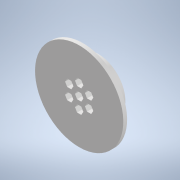
# Autodesk Inventor part: tire vtulka2
Saved by Autodesk Inventor 2022 (Build 260153000, 153)
## iProperties
Created: 2023-02-08
Part Number: tire vtulka2
Material: Типовые
Document SubType Name: Modeling
Designer: akapu
Density: 1 g/cm^3
Appearance: По умолчанию
Author: akapu
Autodesk Inventor part; units mm, degrees
ref_plane "YZ Plane" through (0, 0, 0) normal (1, 0, 0) x (0, 1, 0)
ref_plane "XZ Plane" through (0, 0, 0) normal (0, 1, 0) x (-1, 0, 0)
ref_plane "XY Plane" through (0, 0, 0) normal (0, 0, 1) x (1, 0, 0)
sketch "Эскиз1" plane through (0, 0, 0) normal (1, 0, 0) x (0, 1, 0)
  line L0 (-3.98, -3) -> (-3.38, 0)
  line L1 (-3.98, -3) -> (-56.02, -3) projected
  line L2 (-4.48, -22.93) -> (-4.48, -3)
  line L3 (-55.52, -22.93) -> (-55.52, -3)
  line L4 (-3.98, -3) -> (-56.02, -3) projected
  line L5 (-56.02, -3) -> (-56.62, 0)
  line L6 (-60, 0) -> (0, 0) projected
  line L7 (-60, 0) -> (-60, -22.93)
  line L8 (0, 0) -> (0, -22.93)
  line L9 (-60, -22.93) -> (0, -22.93) projected
  line L10 (-3.98, -3) -> (-3.98, -3)
  line L11 (-3.98, -3) -> (-3.38, 0)
  line L12 (-56.02, -3) -> (-56.02, -3)
  line L13 (-56.02, -3) -> (-56.62, 0)
  line L14 (-3.38, 0) -> (4.62, 0)
  line L15 (-56.62, 0) -> (-64.62, 0)
  line L16 (-64.62, 0) -> (-64.62, 3)
  line L17 (-64.62, 3) -> (4.62, 3)
  line L18 (4.62, 3) -> (4.62, 0)
  line L19 (-30, -3) -> (-51.25, -3)
  line L20 (-51.25, -3) -> (-8.75, -3)
  line L21 (-8.75, -3) -> (-8.75, -22.93)
  line L22 (-51.25, -3) -> (-51.25, -22.93)
  line L23 (-52.5, -22.93) -> (-51.25, -22.93)
  line L24 (-51.5625, -21.93) -> (-51.5625, -22.93)
  line L25 (-51.875, -21.93) -> (-51.25, -21.93)
  line L26 (-52.5, -22.93) -> (-51.25, -20.93)
  spline S0 degree 2 poles (-52.5, -22.93) (-51.1297, -22.7543) (-51.25, -20.93) knots 0 0 0 1 1 1
  line L27 (-8.75, -19) -> (-8.75, -12)
  line L28 (-8.75, -12) -> (-51.25, -12)
  line L29 (-30, 3) -> (-30, -22.93)
  line L30 (-8.75, -12) -> (-11.75, -12)
  line L31 (-30, -12) -> (-30, -14)
  line L32 (-11.75, -12) -> (-13.75, -14)
  line L33 (-11.75, -12) -> (-8.9216, -12) construction
  line L34 (-13.75, -14) -> (-30, -14)
  line L35 (2, 0) -> (0, 0)
  line L36 (-7.75, -4.6) -> (-8.75, -4.6)
  line L37 (-8.25, -4.6) -> (-8.25, -3)
  line L38 (-6.75, -3) -> (-8.75, -3)
  line L39 (-6.75, -3) -> (-8.75, -6.2)
  spline S1 degree 2 poles (-6.75, -3) (-8.9425, -3.2811) (-8.75, -6.2) knots 0 0 0 1 1 1
  spline S2 degree 2 poles (-53.25, -3) (-51.0575, -3.2811) (-51.25, -6.2) knots 0 0 0 1 1 1
  line L40 (-30, -14) -> (-25, -14)
  line L41 (-25, -14) -> (-27, -12)
  point P0 (-51.5625, -22.43)
  point P1 (-30, -15.93)
  point P2 (1.4531, 0)
  point P3 (-8.25, -3.8)
  point P4 (-51.75, -3.8)
  point P5 (-30, -3)
  point P6 (-53.25, -3)
  point P7 (-51.25, -5.3265)
  point P8 (-8.75, -5.3265)
  dimension "d0" = 0
  dimension "d1" = 0
  dimension "d2" = 8
  dimension "d3" = 8
  dimension "d4" = 3
  dimension "d5" = 21.25
  dimension "d6" = 42.5
  dimension "d11" = 7
  dimension "d13" = 3
  dimension "d14" = 2
  dimension "d15" = 135
  dimension "d20" = 0
  dimension "d21" = 0
  dimension "d22" = 9
  dimension "d23" = 5
  constraints: 76 end point, 14 point on line, 7 perpendicular, 6 midpoint, 4 vertical, 3 horizontal, 3 symmetric about line, 1 collinear, 1 equal length, 26 other
  measures "d0" distance of L0.start L10.end
  measures "d1" distance of L1.end L12.end
  measures "d2" distance of L11.end L14.end
  measures "d3" distance of L13.end L15.end
  measures "d4" distance of L15.end L16.end
  measures "d5" distance of L19.start L19.end
  measures "d6" distance of L19.end L20.end
  measures "d11" distance of L27.start L27.end
  measures "d13" distance of L27.end L30.end
  measures "d14" distance of L31.start L31.end
  measures "d15" angle of L32 L33
  measures "d20" distance of L11.end L0.end
  measures "d21" distance of L5.end L13.end
  measures "d22" distance between parallel lines of L20 L28
  measures "d23" distance of L31.end L40.end
revolve "Вращение1" add sketch "Эскиз1" angle 360 about axis through (0, -30, 3) along (0, 0, -1) contours L29 L1 L5 L6 | L6 L15 L16 L17 L29 | L1 L21 S1 L28 L29 | L22 S2 L1 | L28 L32 L34 L41
sketch "Эскиз4" plane through (0, -30, 3) normal (0, 0, 1) x (1, 0, 0)
  line L0 (-1.2721, 9.2093) -> (-2.8003, 12.1239) projected
  line L1 (-2.8003, 12.1239) -> (-1.0404, 14.9046) projected
  line L2 (-1.0404, 14.9046) -> (2.2478, 14.7708) projected
  line L3 (2.2478, 14.7708) -> (3.776, 11.8563) projected
  line L4 (3.776, 11.8563) -> (2.0161, 9.0755) projected
  line L5 (2.0161, 9.0755) -> (-1.2721, 9.2093) projected
  circle A0 centre (0.4878, 11.9901) radius 1.7 projected
  line L6 (-11.8997, 3.6368) -> (-13.428, 6.5513) projected
  line L7 (-13.428, 6.5513) -> (-11.668, 9.3321) projected
  line L8 (-11.668, 9.3321) -> (-8.3798, 9.1983) projected
  line L9 (-8.3798, 9.1983) -> (-6.8516, 6.2837) projected
  line L10 (-6.8516, 6.2837) -> (-8.6116, 3.503) projected
  line L11 (-8.6116, 3.503) -> (-11.8997, 3.6368) projected
  line L12 (-9.0994, -8.4871) -> (-12.3876, -8.3533) projected
  line L13 (-12.3876, -8.3533) -> (-13.9158, -5.4388) projected
  line L14 (-13.9158, -5.4388) -> (-12.1559, -2.658) projected
  line L15 (-12.1559, -2.658) -> (-8.8677, -2.7918) projected
  line L16 (-8.8677, -2.7918) -> (-7.3395, -5.7063) projected
  line L17 (-7.3395, -5.7063) -> (-9.0994, -8.4871) projected
  line L18 (2.8003, -12.1239) -> (1.0404, -14.9046) projected
  line L19 (1.0404, -14.9046) -> (-2.2478, -14.7708) projected
  line L20 (-2.2478, -14.7708) -> (-3.776, -11.8563) projected
  line L21 (-3.776, -11.8563) -> (-2.0161, -9.0755) projected
  line L22 (-2.0161, -9.0755) -> (1.2721, -9.2093) projected
  line L23 (1.2721, -9.2093) -> (2.8003, -12.1239) projected
  line L24 (11.8997, -3.6368) -> (13.428, -6.5513) projected
  line L25 (13.428, -6.5513) -> (11.668, -9.3321) projected
  line L26 (11.668, -9.3321) -> (8.3798, -9.1983) projected
  line L27 (8.3798, -9.1983) -> (6.8516, -6.2837) projected
  line L28 (6.8516, -6.2837) -> (8.6116, -3.503) projected
  line L29 (8.6116, -3.503) -> (11.8997, -3.6368) projected
  line L30 (9.0994, 8.4871) -> (12.3876, 8.3533) projected
  line L31 (12.3876, 8.3533) -> (13.9158, 5.4388) projected
  line L32 (13.9158, 5.4388) -> (12.1559, 2.658) projected
  line L33 (12.1559, 2.658) -> (8.8677, 2.7918) projected
  line L34 (8.8677, 2.7918) -> (7.3395, 5.7063) projected
  line L35 (7.3395, 5.7063) -> (9.0994, 8.4871) projected
  point P0 (0, 30)
extrude "Выдавливание3" cut sketch "Эскиз4" against normal blind 10 contours L0 L1 L2 L3 L4 L5 | A0 | L6 L7 L8 L9 L10 L11 | L12 L13 L14 L15 L16 L17 | L18 L19 L20 L21 L22 L23 | L24 L25 L26 L27 L28 L29 | L30 L31 L32 L33 L34 L35
sketch "Эскиз5" plane through (0, -30, -7) normal (0, 0, 1) x (1, 0, 0)
  circle A0 centre (0.4878, 11.9901) radius 1.7 projected
  circle A1 centre (10.6276, 5.5726) radius 1.7 projected
  circle A2 centre (10.1398, -6.4175) radius 1.7 projected
  circle A3 centre (-0.4878, -11.9901) radius 1.7 projected
  circle A4 centre (-10.6276, -5.5726) radius 1.7 projected
  circle A5 centre (-10.1398, 6.4175) radius 1.7 projected
  point P0 (0, 30)
extrude "Выдавливание4" cut sketch "Эскиз5" against normal blind 10
sketch "Эскиз6" plane through (0, -30, 3) normal (0, 0, 1) x (1, 0, 0)
  circle A0 centre (0, 0) radius 3
  point P0 (0, 30)
  dimension "d28" = 6
  constraints: 1 centre point
  measures "d28" diameter of A0
extrude "Выдавливание5" cut sketch "Эскиз6" against normal blind 20
sketch "Эскиз7" plane through (0, -30, -14) normal (0, 0, -1) x (-1, 0, 0)
  line L0 (0, 0) -> (0, 4.2)
  line L1 (2.4249, 4.2) -> (4.8497, 0)
  line L2 (4.8497, 0) -> (2.4249, -4.2)
  line L3 (2.4249, -4.2) -> (-2.4249, -4.2)
  line L4 (-2.4249, -4.2) -> (-4.8497, 0)
  line L5 (-4.8497, 0) -> (-2.4249, 4.2)
  line L6 (-2.4249, 4.2) -> (2.4249, 4.2)
  point P0 (0, 30)
  dimension "d31" = 4.2
  constraints: 14 end point, 1 coincident, 1 midpoint, 1 vertical, 13 other
  measures "d31" distance of L0.start L0.end
extrude "Выдавливание6" cut sketch "Эскиз7" against normal blind 8
